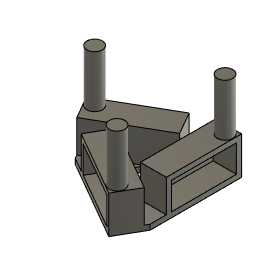
Bottom3 v2 (Autodesk Fusion 360 design; units mm, degrees)
Autodesk Fusion 360 part; units mm, degrees
note: some values were not read from the file. Set by a fixed rule: which sketch regions a step uses.
sketch "草图1" plane through (0, 0, 0) normal (0, 1, 0) x (1, 0, 0)
  circle A0 centre (0, 0) radius 6
  line L0 (7, 0) -> (7, -6)
  line L1 (7, 0) -> (7, 19)
  line L2 (7, 19) -> (16, 19)
  line L3 (16, 19) -> (16, 21)
  line L4 (16, 21) -> (6, 21)
  line L5 (6, 21) -> (6, -8)
  line L6 (6, -8) -> (16, -8)
  line L7 (16, -8) -> (16, -6)
  line L8 (16, -6) -> (7, -6)
  line L9 (-24.4545, 4.3564) -> (-26.1865, 3.3564)
  line L10 (-26.1865, 3.3564) -> (-21.1865, -5.3038)
  line L11 (-19.9545, -3.4378) -> (-24.4545, 4.3564)
  line L12 (-2.8038, 16.8564) -> (1.6962, 9.0622)
  line L13 (-1.0718, 17.8564) -> (-2.8038, 16.8564)
  line L14 (-3.5, 6.0622) -> (1.6962, 9.0622)
  line L15 (3.9282, 9.1962) -> (-1.0718, 17.8564)
  line L16 (-3.5, 6.0622) -> (-19.9545, -3.4378)
  line L17 (-21.1865, -5.3038) -> (3.9282, 9.1962)
  line L18 (8.4545, -23.3564) -> (10.1865, -24.3564)
  line L19 (10.1865, -24.3564) -> (15.1865, -15.6962)
  line L20 (12.9545, -15.5622) -> (8.4545, -23.3564)
  line L21 (-13.1962, -10.8564) -> (-8.6962, -3.0622)
  line L22 (-14.9282, -9.8564) -> (-13.1962, -10.8564)
  line L23 (-3.5, -6.0622) -> (-8.6962, -3.0622)
  line L24 (-9.9282, -1.1962) -> (-14.9282, -9.8564)
  line L25 (-3.5, -6.0622) -> (12.9545, -15.5622)
  line L26 (15.1865, -15.6962) -> (-9.9282, -1.1962)
  dimension "d1" = 12
  dimension "d2" = 6
  dimension "d3" = 19
  dimension "d5" = 360
  constraint coincident A0.centre origin
  constraint vertical L0
  constraint parallel L0 L1
  constraint perpendicular L1 L2
  constraint perpendicular L2 L3
  constraint perpendicular L3 L4
  constraint perpendicular L4 L5
  constraint perpendicular L5 L6
  constraint perpendicular L6 L7
  constraint perpendicular L0 L8
  measures "d1" diameter of A0
  measures "d2" distance of L0.start L0.end
  measures "d3" distance of L0.start L1.end
sketch "草图2" plane through (0, 0, 0) normal (0, 1, 0) x (1, 0, 0)
  circle A0 centre (0, 0) radius 6
  line L0 (16, 21) -> (0, 21)
  line L1 (16, 21) -> (16, -15)
  line L2 (-26.1865, 3.3564) -> (-18.1865, -10.5)
  line L3 (-26.1865, 3.3564) -> (4.9904, 21.3564)
  line L4 (10.1865, -24.3564) -> (18.1865, -10.5)
  line L5 (10.1865, -24.3564) -> (-20.9904, -6.3564)
  dimension "d11" = 360
  constraint coincident A0.centre origin
  constraint perpendicular L0 L1
  constraint vertical L1
extrude "拉伸1" add sketch "草图2" against normal blind 2
extrude "拉伸2" add sketch "草图1" along normal blind 10.5 contours L18 L19 L20 L21 L22 L23 L24 L25 L26 | L9 L10 L11 L12 L13 L14 L15 L16 L17 | L0 L1 L2 L3 L4 L5 L6 L7 L8
sketch "草图3" plane through (0, 10.5, 0) normal (0, 1, 0) x (-1, 0, 0)
  line L0 (-7, 6) -> (-7, -19)
  line L1 (-7, -19) -> (-16, -19)
  line L2 (-16, -19) -> (-16, -21)
  line L3 (-16, -21) -> (-6, -21)
  line L4 (-6, -21) -> (-6, 8)
  line L5 (-6, 8) -> (-16, 8)
  line L6 (-16, 8) -> (-16, 6)
  line L7 (-16, 6) -> (-7, 6)
  line L8 (-6, -21) -> (-16, -21)
  line L9 (-16, -21) -> (-16, 8)
  line L10 (-16, 8) -> (-6, 8)
  line L11 (-6, 8) -> (-6, -21)
  line L12 (21.1865, 5.3038) -> (26.1865, -3.3564)
  line L13 (-3.9282, -9.1962) -> (21.1865, 5.3038)
  line L14 (26.1865, -3.3564) -> (1.0718, -17.8564)
  line L15 (1.0718, -17.8564) -> (-3.9282, -9.1962)
  line L16 (-15.1865, 15.6962) -> (-10.1865, 24.3564)
  line L17 (9.9282, 1.1962) -> (-15.1865, 15.6962)
  line L18 (-10.1865, 24.3564) -> (14.9282, 9.8564)
  line L19 (14.9282, 9.8564) -> (9.9282, 1.1962)
  dimension "d13" = 360
  constraint horizontal L8
  constraint vertical L9
  constraint horizontal L10
  constraint vertical L11
  constraint coincident L5.end L6.start
  constraint coincident L3.end L4.start
extrude "拉伸3" add sketch "草图3" along normal blind 2
cylinder "圆柱体基本要素1" add diameter 6 height 20 placed x (1, 0, 0) y (0, 0, -1) z (0, 1, 0) at (9, 12.5, 20)
pattern_circular "C-阵列1" count 3 over 360 about axis through (0, 1.75, 0) along (0, 1, 0) of "圆柱体基本要素1"
